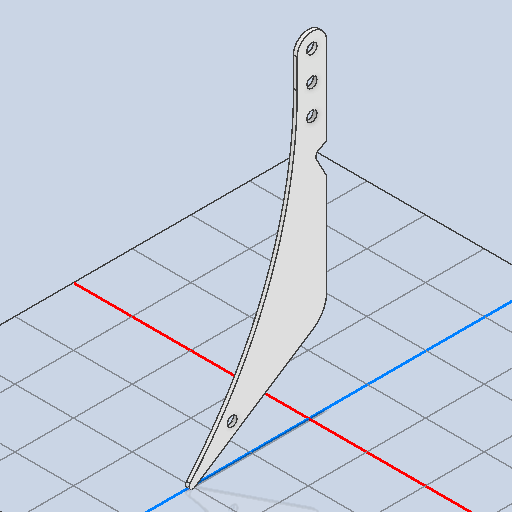
# Autodesk Inventor part: Ramp
Saved by Autodesk Inventor 2026 (Build 300175000, 175)
## iProperties
Created: 2025-04-08
Part Number: Ramp
Material: Acetal Resin, White
Document SubType Name: Modeling
Designer: avere
Density: 1.425 g/cm^3
Appearance: Smooth - White
Author: avere
Autodesk Inventor part; units mm, degrees
ref_plane "YZ Plane" through (0, 0, 0) normal (1, 0, 0) x (0, 1, 0)
ref_plane "XZ Plane" through (0, 0, 0) normal (0, 1, 0) x (-1, 0, 0)
ref_plane "XY Plane" through (0, 0, 0) normal (0, 0, 1) x (1, 0, 0)
sketch "main" plane through (0, 0, 0) normal (0, 0, 1) x (1, 0, 0)
  circle A0 centre (44.478, -90.8155) radius 2.1844
  circle A1 centre (57.178, -90.8155) radius 2.1844
  arc A2 (57.178, -97.1655) -> (57.178, -84.4655) centre (57.178, -90.8155) ccw
  line L0 (57.178, -84.4655) -> (44.478, -84.4655)
  arc A3 (-79.5649, -38.0785) -> (44.478, -84.4655) centre (44.478, 104.579) ccw
  line L1 (57.178, -97.1655) -> (-37.5752, -97.1655)
  line L2 (-48.185, -91.4456) -> (-81.9328, -40.149)
  arc A4 (-79.5649, -38.0785) -> (-81.9328, -40.149) centre (-80.6066, -39.2765) ccw
  arc A5 (-48.185, -91.4456) -> (-37.5752, -97.1655) centre (-37.5752, -84.4655) ccw
  circle A6 centre (31.778, -90.8155) radius 2.1844
  point P0 (7.1274, -71.1865)
  point P1 (-89.2204, -29.0719)
  point P2 (-44.422, -97.1655)
  dimension "d1" = 12.7
  dimension "d2" = 101.6
  dimension "d3" = 1.5875
  dimension "d4" = 12.7
  dimension "d7" = 61.4024
  dimension "d10" = 12.7
  measures "d1" diameter of A2
  measures "d2" distance of L1.start point (-44.422, -97.166)
  measures "d3" radius of A4
  measures "d4" radius of A5
  measures "d7" distance of L2.start L2.end
  measures "d10" distance of A0.centre A6.centre
sketch "Sketch1" plane through (0, 0, 0) normal (1, 0, 0) x (0, 1, 0)
  arc A0 (-39.5025, -3.0335) -> (-42.7248, -2.0551) centre (-41.6029, -4.1554) ccw projected
  line L0 (-42.7248, -2.0551) -> (-52.3306, -7.186) projected
  line L1 (-39.5025, -3.0335) -> (-35.7298, -10.0964) projected
  circle A1 centre (-122.5435, 34.4996) radius 2.0955
  circle A2 centre (-12.7, 0) radius 2.1844
  circle A3 centre (0, 0) radius 2.1844
  arc A4 (0, -6.35) -> (0, 6.35) centre (0, 0) ccw
  line L2 (0, 6.35) -> (-12.7, 6.35)
  arc A5 (-136.743, 52.737) -> (-12.7, 6.35) centre (-12.7, 195.3946) ccw
  line L3 (0, -6.35) -> (-94.7533, -6.35)
  line L4 (-105.3631, -0.6301) -> (-139.1109, 50.6665)
  arc A6 (-136.743, 52.737) -> (-139.1109, 50.6665) centre (-137.7846, 51.539) ccw
  arc A7 (-105.3631, -0.6301) -> (-94.7533, -6.35) centre (-94.7533, 6.35) ccw
  circle A8 centre (-25.4, 0) radius 2.1844
  point P0 (-50.7654, -6.35)
  point P1 (-37.731, -6.35)
  constraints: 1 centre point, 3 other
extrude "Extrusion1" add sketch "Sketch1" along normal blind 1.5875 contours A0 L0 L3 A7 L4 A6 A5 L2 A4 L1
body "Solid1"
